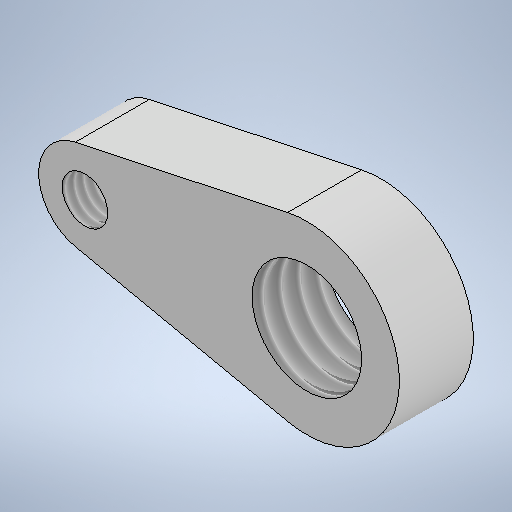
# Autodesk Inventor part: 214.1
Saved by Autodesk Inventor 2025 (Build 290162010, 162A)
## iProperties
Created: 2024-06-09
Part Number: 214.1
Material: Generic
Document SubType Name: Modeling
Designer: Fabri
Density: 1 g/cm^3
Appearance: Default
Author: Fabri
Autodesk Inventor part; units mm, degrees
ref_plane "YZ Plane" through (0, 0, 0) normal (1, 0, 0) x (0, 1, 0)
ref_plane "XZ Plane" through (0, 0, 0) normal (0, 1, 0) x (-1, 0, 0)
ref_plane "XY Plane" through (0, 0, 0) normal (0, 0, 1) x (1, 0, 0)
sketch "Sketch1" plane through (0, 0, 0) normal (0, 1, 0) x (-1, 0, 0)
  arc A0 (12.5208, -2.4451) -> (12.5208, 2.4451) centre (12, 0) ccw
  arc A1 (1.0417, 4.8903) -> (1.0417, -4.8903) centre (0, 0) ccw
  line L0 (1.0417, 4.8903) -> (12.5208, 2.4451)
  line L1 (12.5208, -2.4451) -> (1.0417, -4.8903)
  dimension "d0" = 2.5
  dimension "d1" = 5
  dimension "d2" = 12
  constraints: 4 end point, 4 point on circle, 4 tangent, 2 centre point, 2 coincident, 1 horizontal alignment
  measures "d0" radius of A0
  measures "d1" radius of A1
  measures "d2" distance of A1.centre A0.centre
extrude "Extrusion1" add sketch "Sketch1" along normal blind 4
sketch "Sketch3" plane through (0, 4, 0) normal (0, 1, 0) x (1, 0, 0)
  arc A0 (-12.5208, 2.4451) -> (-12.5208, -2.4451) centre (-12, 0) ccw projected
  point P0 (0, 0)
  constraints: 1 coincident
hole "Hole2" at (-12, 4, 0) direction (0, -1, 0) diameter 2.459 end through all thread size "M3x0.5" class "6H" standard "ISO Metric profile"
sketch "Sketch4" plane through (0, 4, 0) normal (0, 1, 0) x (1, 0, 0)
  arc A0 (-1.0417, -4.8903) -> (-1.0417, 4.8903) centre (0, 0) ccw projected
  constraints: 1 coincident
hole "Hole3" at (0, 4, 0) direction (0, -1, 0) diameter 5.9175 end through all thread size "M7x1" class "6H" standard "ISO Metric profile"
body "Solid1"
